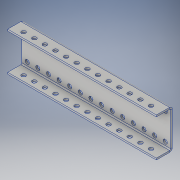
# Autodesk Inventor part: Intake side inner
Saved by Autodesk Inventor 2019 (Build 230136000, 136)
## iProperties
Created: 2018-11-07
Part Number: Intake side inner
Material: Aluminum 6061
Document SubType Name: Sheet Metal
Designer: woodk
Density: 2.7 g/cm^3
Sheet Metal Rule: Haakon
Appearance: Aluminum - Flat
Mass: 74.1007 g
Surface Area: 288.817 cm^2
Volume: 27.4447 cm^3
Author: woodk
Autodesk Inventor part; units mm, degrees
ref_plane "YZ Plane" through (0, 0, 0) normal (1, 0, 0) x (0, 1, 0)
ref_plane "XZ Plane" through (0, 0, 0) normal (0, 1, 0) x (-1, 0, 0)
ref_plane "XY Plane" through (0, 0, 0) normal (0, 0, 1) x (1, 0, 0)
sketch "Sketch1" plane through (0, 0, 0) normal (0, 0, 1) x (1, 0, 0)
  line L0 (0, 0) -> (177.8, 0)
  line L1 (177.8, 0) -> (177.8, 46.736)
  line L2 (177.8, 46.736) -> (0, 46.736)
  line L3 (0, 46.736) -> (0, 0)
  dimension "d0" = 46.736
  dimension "d1" = 177.8
  measures "d0" distance of L2.end L0.start
  measures "d1" distance of L0.start L0.end
extrude "Plate1" add sketch "Sketch1" along normal blind 2.032
sketch "Sketch2" plane through (0, 44.704, 0) normal (0, 1, 0) x (-1, 0, 0)
  line L0 (-177.8, 0) -> (0, 0)
  line L1 (0, 0) -> (0, 19.05)
  line L2 (0, 19.05) -> (-177.8, 19.05)
  line L3 (-177.8, 19.05) -> (-177.8, 0)
  constraints: 6 end point, 1 horizontal, 1 perpendicular, 1 vertical
edge flange "Flange1" height 19.05 angle 90 thickness 2.032 bend radius 1.27 thickness toward (0, 1, 0) relief tear relief width 2.032 relief depth 1.016 edges at (88.9, 46.736, 2.032) wall of the first edge with corners at (177.8, 44.704, 0) (0, 44.704, 0) (0, 44.704, 19.05) (177.8, 44.704, 19.05)
bend "Bend1"
corner "Corner1"
sketch "Sketch3" plane through (177.8, 2.032, 0) normal (0, -1, 0) x (1, 0, 0)
  line L0 (-177.8, 0) -> (0, 0)
  line L1 (0, 0) -> (0, 19.05)
  line L2 (0, 19.05) -> (-177.8, 19.05)
  line L3 (-177.8, 19.05) -> (-177.8, 0)
  constraints: 6 end point, 1 horizontal, 1 perpendicular, 1 vertical
edge flange "Flange2" height 19.05 angle 90 thickness 2.032 bend radius 1.27 thickness toward (0, -1, 0) relief tear relief width 2.032 relief depth 1.016 edges at (88.9, 0, 2.032) wall of the first edge with corners at (0, 2.032, 0) (177.8, 2.032, 0) (177.8, 2.032, 19.05) (0, 2.032, 19.05)
bend "Bend2"
corner "Corner2"
sketch "Sketch4" plane through (0, 46.736, 19.05) normal (0, 1, 0) x (1, 0, 0)
  line L0 (0, 0) -> (0, 15.748) projected
  line L1 (0, 19.05) -> (177.8, 19.05) projected
  point P0 (12.7, 6.35)
  dimension "d23" = 12.7
  dimension "d24" = 12.7
  measures "d23" distance from line of L0 point (12.7, 6.35)
  measures "d24" distance from line of L1 point (12.7, 6.35)
hole "Hole1" at (12.7, 46.736, 12.7) direction (0, -1, 0) diameter 4.9784 end through all
pattern_linear "Rectangular Pattern1" count 13 spacing 12.7 along (1, 0, 0) of "Hole1"
sketch "Sketch5" plane through (0, 0, 0) normal (0, 0, -1) x (-1, 0, 0)
  line L0 (-177.8, 3.302) -> (-177.8, 43.434) projected
  line L1 (-177.8, 46.736) -> (0, 46.736) projected
  line L2 (0, 0) -> (-177.8, 0) projected
  point P0 (-171.45, 39.243)
  point P1 (-171.45, 7.493)
  dimension "d35" = 6.35
  dimension "d36" = 7.493
  dimension "d37" = 7.493
  constraints: 1 vertical alignment
  measures "d35" distance from line of L0 point (-171.45, 39.243)
  measures "d36" distance from line of L1 point (-171.45, 39.243)
  measures "d37" distance from line of L2 point (-171.45, 7.493)
hole "Hole2" at (171.45, 39.243, 0) at (171.45, 7.493, 0) direction (0, 0, 1) diameter 4.9784 end through all
pattern_linear "Rectangular Pattern2" count 14 spacing 12.7 along (-1, 0, 0) of "Hole2"
equation "\"d30\" = Thickness"
equation "\"d37\" = d36"
equation "\"d43\" = Thickness"
equation "\"d2\" = Thickness"
equation "\"d3\" = BendReliefWidth"
equation "\"d4\" = BendReliefDepth"
equation "\"d5\" = MinimumRemnant"
equation "\"d6\" = TransitionRadius"
equation "\"d9\" = BendRadius"
equation "\"d10\" = CornerReliefSize"
equation "\"d11\" = GapSize"
equation "\"d12\" = JacobiRadiusSize"
equation "\"d13\" = BendReliefWidth"
equation "\"d14\" = BendReliefDepth"
equation "\"d15\" = MinimumRemnant"
equation "\"d16\" = TransitionRadius"
equation "\"d19\" = BendRadius"
equation "\"d20\" = CornerReliefSize"
equation "\"d21\" = GapSize"
equation "\"d22\" = JacobiRadiusSize"
equation "\"BendReliefWidth\" = Thickness"
equation "\"BendReliefDepth\" = 0.5 * Thickness"
equation "\"CornerReliefSize\" = 4 * Thickness"
equation "\"MinimumRemnant\" = 2 * Thickness"
equation "\"TransitionRadius\" = BendRadius"
equation "\"JacobiRadiusSize\" = BendRadius"
equation "\"GapSize\" = Thickness"
equation "\"Thickness\" = 2.032"
equation "\"BendRadius\" = 1.27"
body "Solid1"
